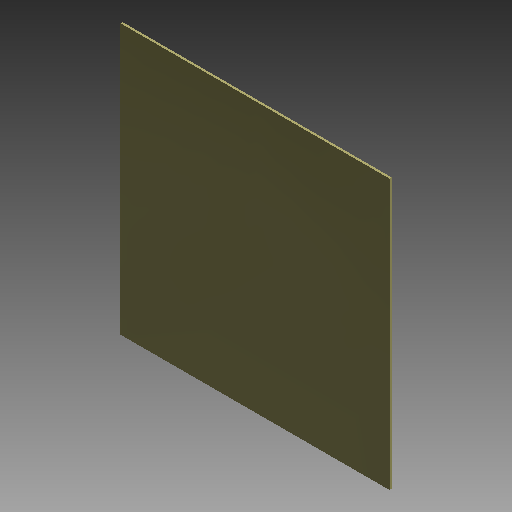
# Autodesk Inventor part: TestPoint
Saved by Autodesk Inventor 2018.2 (Build 222227000, 227)
## iProperties
Part Number: TestPoint
Material: Generic
Document SubType Name: Modeling
Designer: autocad
Appearance: TP1-27, TestPoint
Author: autocad
Autodesk Inventor part; units mm, degrees
ref_plane "YZ Plane" through (0, 0, 0) normal (1, 0, 0) x (0, 1, 0)
ref_plane "XZ Plane" through (0, 0, 0) normal (0, 1, 0) x (-1, 0, 0)
ref_plane "XY Plane" through (0, 0, 0) normal (0, 0, 1) x (1, 0, 0)
sketch "TP1-27, TestPoint_13" plane through (0, 0, 0) normal (0, 0, 1) x (1, 0, 0)
  line L0 (-0.64, -0.6387) -> (0.6349, -0.6387)
  line L1 (0.6349, -0.6387) -> (0.6349, 0.6388)
  line L2 (0.6349, 0.6388) -> (-0.64, 0.6388)
  line L3 (-0.64, 0.6388) -> (-0.64, -0.6387)
  constraints: 8 end point
extrude "Extrusion1" add sketch "TP1-27, TestPoint_13" along normal blind 0.01
body "Solid1"
